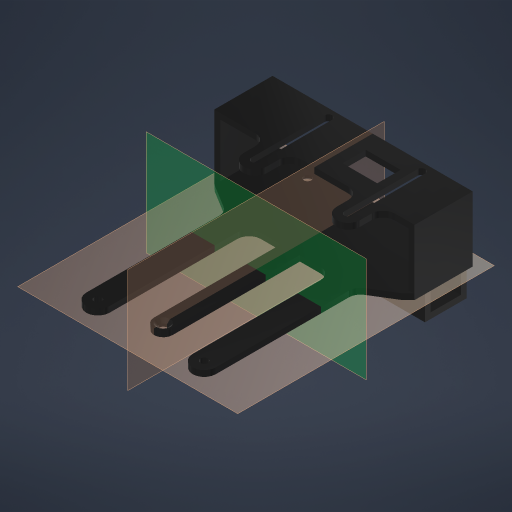
# Autodesk Inventor part: PD_Main
Saved by Autodesk Inventor 2024 (Build 280153000, 153)
## iProperties
Manager: Louis Van Roosmaelen
Company: DCS - DIGITAL COMBAT SIMULATOR
Created: 2023-12-17
Part Number: PD_Main
Material: S235
Catalog Web Link: http://emmausbovenbouw.op-weg.be/
Vendor: Emmaüsinstituut Bovenbouw Aalter
Document SubType Name: Modeling
Designer: Louis
Engineer: Declercq St.
Manufacturer: Standard
Standards Organization: Custom
Density: 7.86 g/cm^3
Appearance: Smooth - Black
Mass: 188.232 g
Surface Area: 215.295 cm^2
Volume: 23.9481 cm^3
IDENT.NR.: AJ2022
TEAM: 30
Title: F18C Home Cockpit
Author: Louis
Keywords: Ø
Autodesk Inventor part; units mm, degrees
sketch "Sketch1" plane through (0, 0, 0) normal (0, 0, 1) x (1, 0, 0)
  line L0 (0, 2.8582) -> (0, -2.8582) construction
  line L1 (-5.7775, 0) -> (5.7775, 0) construction
  line L2 (-40.5, -50) -> (40.5, -50)
  line L3 (40.5, -50) -> (40.5, 50)
  line L4 (40.5, 50) -> (-40.5, 50)
  line L5 (-40.5, 50) -> (-40.5, -50)
  line L6 (-40.5, -50) -> (40.5, 50) construction
  line L7 (40.5, -50) -> (-40.5, 50) construction
  line L8 (-43, 52.5) -> (43, 52.5)
  line L9 (43, 52.5) -> (43, -52.5)
  line L10 (43, -52.5) -> (-43, -52.5)
  line L11 (-43, -52.5) -> (-43, 52.5)
  line L12 (-43, 52.5) -> (43, -52.5) construction
  line L13 (43, 52.5) -> (-43, -52.5) construction
  point P0 (0, 0)
  point P1 (0, 0)
  dimension "d0" = 81
  dimension "d1" = 100
  dimension "d2" = 2.5
  dimension "d3" = 2.5
  constraints: 28 end point, 6 midpoint, 4 parallel, 3 horizontal, 2 perpendicular, 1 coincident, 1 vertical
  measures "d0" distance of L4.end L3.end
  measures "d1" distance of L3.end L2.end
  measures "d2" distance between parallel lines of L3 L9
  measures "d3" distance between parallel lines of L10 L2
extrude "Extrusion1" add sketch "Sketch1" along normal blind 2.5 contours L5 L4 L3 L2
sketch "Sketch2" plane through (0, 0, 0) normal (0, 0, -1) x (-1, 0, 0)
  line L0 (40.5, -50) -> (-40.5, -50) projected
  line L1 (-40.5, -50) -> (-40.5, 50) projected
  line L2 (-40.5, 50) -> (40.5, 50) projected
  line L3 (40.5, 50) -> (40.5, -50) projected
  line L4 (-40.5, 50) -> (-13, 50)
  line L5 (-13, 50) -> (-13, 32)
  line L6 (-13, 32) -> (-40.5, 32)
  line L7 (-40.5, 32) -> (-40.5, 50)
  line L8 (-40.5, 34.5) -> (-15.5, 34.5)
  line L9 (-15.5, 34.5) -> (-15.5, 47.5)
  line L10 (-15.5, 47.5) -> (-40.5, 47.5)
  point P0 (0, 0)
  dimension "d6" = 27.5
  dimension "d7" = 18
  dimension "d8" = 2.5
  dimension "d9" = 2.5
  dimension "d10" = 2.5
  constraints: 14 end point, 3 perpendicular, 2 parallel, 2 point on line, 1 horizontal, 1 vertical
  measures "d6" distance of L5.end L6.end
  measures "d7" distance of L4.end L5.end
  measures "d8" distance between parallel lines of L2 L10
  measures "d9" distance between parallel lines of L6 L8
  measures "d10" distance between parallel lines of L5 L9
extrude "Extrusion2" add sketch "Sketch2" along normal blind 13 contours L1 L8 L9 L10 L2 L5 L6
sketch "Sketch3" plane through (0, 0, -13) normal (0, 0, -1) x (-1, 0, 0)
  line L0 (-13, 50) -> (-13, 32) projected
  line L1 (-13, 32) -> (-40.5, 32) projected
  line L2 (-40.5, 32) -> (-40.5, 34.5) projected
  line L3 (-40.5, 34.5) -> (-15.5, 34.5) projected
  line L4 (-15.5, 34.5) -> (-15.5, 47.5) projected
  line L5 (-15.5, 47.5) -> (-40.5, 47.5) projected
  line L6 (-40.5, 47.5) -> (-40.5, 50) projected
  line L7 (-40.5, 50) -> (-13, 50) projected
  line L8 (-40.5, 34.5) -> (-40.5, 47.5) projected
  line L9 (-40.5, 34.5) -> (-40.5, 47.5)
  point P0 (0, 0)
  constraints: 2 end point, 1 vertical
extrude "Extrusion3" add sketch "Sketch3" against normal blind 2.5 contours L5 L4 L3 L8
sketch "Sketch4" plane through (13, 32, 0) normal (-1, 0, 0) x (0, 0, 1)
  line L0 (0, 18) -> (0, 0) projected
  line L1 (0, 0) -> (-13, 0) projected
  line L2 (-13, 0) -> (-13, 18) projected
  line L3 (-13, 18) -> (0, 18) projected
  line L4 (0, 18) -> (2.5, 18) projected
  line L5 (2.5, 18) -> (2.5, -82) projected
  line L6 (2.5, -82) -> (0, -82) projected
  line L7 (0, -82) -> (0, 0) projected
  point P0 (0, -32)
  point P1 (-5.25, 11)
  point P2 (-5.25, 7)
  dimension "d15" = 7
  dimension "d16" = 4
  dimension "d19" = 5.25
  dimension "d20" = 5.25
  measures "d15" distance from line of point (-5.25, 7) L1
  measures "d16" distance of point (-5.25, 7) point (-5.25, 11)
  measures "d19" distance from line of L0 point (-5.25, 7)
  measures "d20" distance from line of L0 point (-5.25, 11)
hole "Hole1" at (13, 43, -5.25) at (13, 39, -5.25) direction (1, 0, 0) diameter 4 end through all counterbore diameter 8 counterbore depth 4
sketch "Sketch6" plane through (40.5, -50, 2.5) normal (1, 0, 0) x (0, 0, -1)
  line L0 (13, 84.5) -> (13, 97.5) projected
  line L1 (13, 97.5) -> (2.5, 97.5) projected
  line L2 (2.5, 97.5) -> (2.5, 84.5) projected
  line L3 (2.5, 84.5) -> (13, 84.5) projected
  line L4 (15.5, 82) -> (2.5, 82) projected
  line L5 (2.5, 82) -> (2.5, 0) projected
  line L6 (2.5, 0) -> (0, 0) projected
  line L7 (0, 0) -> (0, 100) projected
  line L8 (0, 100) -> (15.5, 100) projected
  line L9 (15.5, 100) -> (15.5, 82) projected
  line L10 (2.5, 100) -> (2.5, 82) projected
  line L11 (2.5, 100) -> (-25.5, 100)
  line L12 (-25.5, 100) -> (-25.5, 75)
  line L13 (-25.5, 75) -> (2.5, 75)
  line L14 (2.5, 75) -> (2.5, 100)
  point P0 (2.5, 50)
  dimension "d32" = 28
  dimension "d33" = 25
  constraints: 8 end point, 2 parallel, 1 horizontal, 1 perpendicular
  measures "d32" distance of L13.end L12.end
  measures "d33" distance of L12.end L11.end
extrude "Extrusion5" add sketch "Sketch6" along normal blind 2.5 contours L10 L5 L13 L7 L8 L2 | L7 L13 L12 L11
mirror "Mirror2" about plane through (0, 0, 0) normal (1, 0, 0) of "Extrusion5", "Hole1", "Extrusion3", "Extrusion2"
sketch "Sketch7" plane through (40.5, 25, 28) normal (0, 0, 1) x (1, 0, 0)
  line L0 (-81, 25) -> (-81, 0) projected
  line L1 (-81, 0) -> (-83.5, 0) projected
  line L2 (-83.5, 0) -> (-83.5, 25) projected
  line L3 (-83.5, 25) -> (-81, 25) projected
  line L4 (0, 0) -> (0, 25) projected
  line L5 (0, 25) -> (2.5, 25) projected
  line L6 (2.5, 25) -> (2.5, 0) projected
  line L7 (2.5, 0) -> (0, 0) projected
  line L8 (0, 0) -> (-81, 0)
  line L9 (-81, 25) -> (0, 25)
  point P0 (-40.5, -25)
  constraints: 4 end point, 1 horizontal, 1 parallel
extrude "Extrusion6" add sketch "Sketch7" against normal blind 2.5 contours L9 L4 L8 L0
chamfer "Chamfer1" distance 2.5 angle 45 2 edges at (-40.5, 25, 1.25) (40.5, 25, 1.25)
sketch "Sketch9" plane through (0, 0, 2.5) normal (0, 0, 1) x (1, 0, 0)
  line L0 (-40.5, 22.5) -> (-43, 25) projected
  line L1 (-40.5, 25) -> (-43, 25) projected
  line L2 (-40.5, 50) -> (-40.5, 25) projected
  line L3 (-43, 50) -> (-40.5, 50) projected
  line L4 (-43, 25) -> (-43, 50) projected
  line L5 (-40.5, -50) -> (-40.5, 22.5) projected
  line L6 (40.5, -50) -> (-40.5, -50) projected
  line L7 (40.5, 22.5) -> (40.5, -50) projected
  line L8 (43, 25) -> (40.5, 22.5) projected
  line L9 (43, 50) -> (43, 25) projected
  line L10 (40.5, 50) -> (43, 50) projected
  line L11 (-40.5, 50) -> (40.5, 50) projected
  line L12 (43, 25) -> (40.5, 25) projected
  line L13 (40.5, 25) -> (40.5, 50) projected
  circle A0 centre (-22.86, -45.25) radius 5
  circle A1 centre (22.86, -45.25) radius 5
  line L14 (-27.86, -45.25) -> (-27.86, 14.75)
  line L15 (-27.86, 14.75) -> (-40.5, 22.5)
  line L16 (-17.86, -45.25) -> (-17.86, 14.75)
  line L17 (-17.86, -45.25) -> (42.14, -45.25) construction
  line L18 (17.86, -45.25) -> (17.86, 14.75)
  line L19 (17.86, 14.75) -> (-17.86, 14.75)
  line L20 (27.86, -45.25) -> (27.86, 14.75)
  line L21 (27.86, 14.75) -> (40.5, 22.5)
  point P0 (0, 0)
  point P1 (24.4212, -50)
  point P2 (-21.2988, -50)
  point P3 (21.2988, -50)
  point P4 (-24.4212, -50)
  dimension "d58" = 10
  dimension "d59" = 10
  dimension "d60" = 60
  dimension "d61" = 60
  dimension "d62" = 90
  dimension "d63" = 60
  dimension "d64" = 60
  dimension "d65" = 90
  constraints: 16 end point, 4 point on circle, 3 point on line, 2 centre point, 2 coincident, 2 perpendicular, 2 tangent, 1 horizontal, 1 parallel, 1 vertical
  measures "d58" diameter of A0
  measures "d59" diameter of A1
  measures "d60" distance of L14.start L14.end
  measures "d61" distance of L16.start L16.end
  measures "d62" angle of L17 L16
  measures "d63" distance of L18.start L18.end
  measures "d64" distance of L20.start L20.end
  measures "d65" angle of L17 L20
extrude "Extrusion7" cut sketch "Sketch9" against normal up to surface (2.5 mm away) contours L15 L14 A0 L6 L5 | A0 L16 L19 L18 A1 L6 | A1 L20 L21 L7 L6
sketch "Sketch10" plane through (43, 25, 28) normal (0, 0, 1) x (1, 0, 0)
  line L0 (0, 0) -> (-86, 0) projected
  line L1 (-86, 0) -> (-86, 25) projected
  line L2 (-86, 25) -> (0, 25) projected
  line L3 (0, 25) -> (0, 0) projected
  circle A0 centre (-58.5, -10) radius 1.65
  circle A1 centre (-58.5, 21.5) radius 1.65
  circle A2 centre (-18.5, -10) radius 1.65
  circle A3 centre (-18.5, 21.5) radius 1.65
  line L4 (-60.15, -10) -> (-60.15, 21.5)
  line L5 (-56.85, -10) -> (-56.85, 21.5)
  line L6 (-20.15, -10) -> (-20.15, 21.5)
  line L7 (-16.85, -10) -> (-16.85, 21.5)
  circle A4 centre (-58.5, -10) radius 5
  circle A5 centre (-58.5, 21.5) radius 5
  circle A6 centre (-18.5, 21.5) radius 5
  circle A7 centre (-18.5, -10) radius 5
  line L8 (-63.5, -10) -> (-63.5, 21.5)
  line L9 (-53.5, -10) -> (-53.5, 21.5)
  line L10 (-13.5, 21.5) -> (-13.5, -10)
  line L11 (-23.5, -10) -> (-23.5, 21.5)
  point P0 (-43, -25)
  point P1 (-23.5, 0)
  point P2 (-13.5, 0)
  point P3 (-63.5, 0)
  point P4 (-53.5, 0)
  dimension "d68" = 3.3
  dimension "d69" = 3.3
  dimension "d70" = 3.3
  dimension "d71" = 3.3
  dimension "d74" = 40
  dimension "d75" = 40
  dimension "d76" = 15.5
  dimension "d77" = 24.5
  dimension "d78" = 10
  dimension "d79" = 10
  dimension "d80" = 10
  dimension "d81" = 10
  dimension "d82" = 35
  dimension "d83" = 35
  dimension "d88" = 3.5
  dimension "d89" = 3.5
  constraints: 16 end point, 16 point on circle, 8 centre point, 7 tangent, 4 coincident, 2 vertical, 1 parallel
  measures "d68" diameter of A0
  measures "d69" diameter of A1
  measures "d70" diameter of A2
  measures "d71" diameter of A3
  measures "d74" distance of A1.centre A3.centre
  measures "d75" distance of A2.centre A0.centre
  measures "d76" horizontal distance of point (-43, -25) A1.centre
  measures "d77" horizontal distance of point (-43, -25) A2.centre
  measures "d78" diameter of A4
  measures "d79" diameter of A5
  measures "d80" diameter of A6
  measures "d81" diameter of A7
  measures "d82" distance from line of L2 A0.centre
  measures "d83" distance from line of L2 A2.centre
  measures "d88" distance from line of L2 A1.centre
  measures "d89" distance from line of L2 A3.centre
extrude "Extrusion8" add sketch "Sketch10" against normal up to surface (2.5 mm away) contours L10 A7 L7 L0 | L7 A7 L6 L0 | A7 L6 A2 L7 | L6 A7 L11 L0 | L7 A2 L6 A7 | L9 A4 L5 L0 | L5 A4 L4 L0 | A4 L4 A0 L5 | L4 A4 L8 L0 | L5 A0 L4 A4
extrude "Extrusion9" cut sketch "Sketch10" against normal up to surface (2.5 mm away) contours L7 A7 L6 L0 | L0 L6 A6 L7 | L7 A2 L6 A7 | A6 L6 A3 L7 | A3 | L5 A4 L4 L0 | L0 L4 A5 L5 | A5 L4 A1 L5 | L5 A0 L4 A4 | A1 picked at (-18.4337, -6.1416) picked at (-58.5663, -6.1416)
fillet "Fillet1" radius 5 9 edges at (-17.86, 14.75, 1.25) (17.86, 14.75, 1.25) (27.86, 14.75, 1.25) (-27.86, 14.75, 1.25) (-40.5, 22.5001, 1.25) (29.5, 25, 26.75) (19.5, 25, 26.75) (-10.5, 25, 26.75) (-20.5, 25, 26.75)
sketch "Sketch11" plane through (0, 0, 0) normal (0, 0, -1) x (-1, 0, 0)
  arc A0 (24.4212, -50) -> (27.86, -45.25) centre (22.86, -45.25) ccw projected
  line L0 (24.4212, -50) -> (21.2988, -50) projected
  arc A1 (17.86, -45.25) -> (21.2988, -50) centre (22.86, -45.25) ccw projected
  line L1 (17.86, -45.25) -> (17.86, 9.75) projected
  arc A2 (17.86, 9.75) -> (12.86, 14.75) centre (12.86, 9.75) ccw projected
  line L2 (12.86, 14.75) -> (-12.86, 14.75) projected
  arc A3 (-12.86, 14.75) -> (-17.86, 9.75) centre (-12.86, 9.75) ccw projected
  line L3 (-17.86, 9.75) -> (-17.86, -45.25) projected
  arc A4 (-21.2988, -50) -> (-17.86, -45.25) centre (-22.86, -45.25) ccw projected
  line L4 (-21.2988, -50) -> (-24.4212, -50) projected
  arc A5 (-27.86, -45.25) -> (-24.4212, -50) centre (-22.86, -45.25) ccw projected
  line L5 (-27.86, -45.25) -> (-27.86, 11.9507) projected
  arc A6 (-27.86, 11.9507) -> (-30.2465, 16.2132) centre (-32.86, 11.9507) ccw projected
  line L6 (-30.2465, 16.2132) -> (-40.5, 22.5) projected
  line L7 (-40.5, 22.5) -> (-43, 25) projected
  line L8 (-43, 25) -> (-43, 50) projected
  line L9 (-43, 50) -> (-40.5, 50) projected
  line L10 (-40.5, 50) -> (-13, 50) projected
  line L11 (-13, 32) -> (-13, 50) projected
  line L12 (-40.5, 32) -> (-13, 32) projected
  line L13 (-40.5, 34.5) -> (-40.5, 32) projected
  line L14 (-15.5, 34.5) -> (-40.5, 34.5) projected
  line L15 (-15.5, 47.5) -> (-15.5, 34.5) projected
  line L16 (-40.5, 47.5) -> (-15.5, 47.5) projected
  line L17 (-40.5, 50) -> (-40.5, 47.5) projected
  line L18 (27.86, 11.9507) -> (27.86, -45.25) projected
  arc A7 (30.2465, 16.2132) -> (27.86, 11.9507) centre (32.86, 11.9507) ccw projected
  line L19 (39.996, 22.191) -> (30.2465, 16.2132) projected
  arc A8 (39.996, 22.191) -> (40.918, 22.918) centre (37.3825, 26.4536) ccw projected
  line L20 (43, 25) -> (40.918, 22.918) projected
  line L21 (43, 50) -> (43, 25) projected
  line L22 (40.5, 50) -> (43, 50) projected
  line L23 (13, 50) -> (40.5, 50) projected
  line L24 (13, 50) -> (13, 32) projected
  line L25 (13, 32) -> (40.5, 32) projected
  line L26 (40.5, 32) -> (40.5, 34.5) projected
  line L27 (40.5, 34.5) -> (15.5, 34.5) projected
  line L28 (15.5, 34.5) -> (15.5, 47.5) projected
  line L29 (15.5, 47.5) -> (40.5, 47.5) projected
  line L30 (40.5, 47.5) -> (40.5, 50) projected
  line L31 (-13, 50) -> (13, 50) projected
  point P0 (0, 0)
  point P1 (-22.86, 44.92)
  point P2 (22.86, 44.92)
  dimension "d106" = 90.17
  dimension "d107" = 90.17
  dimension "d108" = 45.72
  dimension "d109" = 45.72
  dimension "d110" = 45.72
  constraints: 2 coincident
  measures "d106" distance of point (-22.86, -45.25) point (-22.86, 44.92)
  measures "d107" distance of point (22.86, -45.25) point (22.86, 44.92)
  measures "d108" distance of point (22.86, 44.92) point (-22.86, 44.92)
  measures "d109" distance of point (22.86, -45.25) point (-22.86, -45.25)
  measures "d110" horizontal distance of A0.centre point (-22.86, 44.92)
hole "Hole3" at (22.86, 44.92, 0) at (-22.86, 44.92, 0) direction (0, 0, 1) diameter 3.3 depth 2.5 countersink diameter 6 countersink angle 90
sketch "Sketch12" plane through (0, 0, 0) normal (0, 0, -1) x (-1, 0, 0)
  arc A0 (-24.3909, 47.5) -> (-21.3291, 47.5) centre (-22.86, 44.92) ccw projected
  arc A1 (-24.3909, 47.5) -> (-21.3291, 47.5) centre (-22.86, 44.92) ccw projected
  arc A2 (-21.3291, 47.5) -> (-24.3909, 47.5) centre (-22.86, 44.92) ccw projected
  circle A3 centre (-22.86, 44.92) radius 1.65 projected
  arc A4 (21.3291, 47.5) -> (24.3909, 47.5) centre (22.86, 44.92) ccw projected
  arc A5 (24.3909, 47.5) -> (21.3291, 47.5) centre (22.86, 44.92) ccw projected
  circle A6 centre (22.86, 44.92) radius 1.65 projected
  arc A7 (24.4212, -50) -> (27.86, -45.25) centre (22.86, -45.25) ccw projected
  line L0 (24.4212, -50) -> (21.2988, -50) projected
  arc A8 (17.86, -45.25) -> (21.2988, -50) centre (22.86, -45.25) ccw projected
  line L1 (17.86, -45.25) -> (17.86, 9.75) projected
  arc A9 (17.86, 9.75) -> (12.86, 14.75) centre (12.86, 9.75) ccw projected
  line L2 (12.86, 14.75) -> (-12.86, 14.75) projected
  arc A10 (-12.86, 14.75) -> (-17.86, 9.75) centre (-12.86, 9.75) ccw projected
  line L3 (-17.86, 9.75) -> (-17.86, -45.25) projected
  arc A11 (-21.2988, -50) -> (-17.86, -45.25) centre (-22.86, -45.25) ccw projected
  line L4 (-21.2988, -50) -> (-24.4212, -50) projected
  arc A12 (-27.86, -45.25) -> (-24.4212, -50) centre (-22.86, -45.25) ccw projected
  line L5 (-27.86, -45.25) -> (-27.86, 11.9507) projected
  arc A13 (-27.86, 11.9507) -> (-30.2465, 16.2132) centre (-32.86, 11.9507) ccw projected
  line L6 (-30.2465, 16.2132) -> (-40.5, 22.5) projected
  line L7 (-40.5, 22.5) -> (-43, 25) projected
  line L8 (-43, 25) -> (-43, 50) projected
  line L9 (-43, 50) -> (-40.5, 50) projected
  line L10 (-40.5, 50) -> (-13, 50) projected
  line L11 (-13, 32) -> (-13, 50) projected
  line L12 (-40.5, 32) -> (-13, 32) projected
  line L13 (-40.5, 34.5) -> (-40.5, 32) projected
  line L14 (-15.5, 34.5) -> (-40.5, 34.5) projected
  line L15 (-15.5, 47.5) -> (-15.5, 34.5) projected
  line L16 (-21.3291, 47.5) -> (-15.5, 47.5) projected
  arc A14 (-21.3291, 47.5) -> (-24.3909, 47.5) centre (-22.86, 44.92) ccw projected
  line L17 (-40.5, 47.5) -> (-24.3909, 47.5) projected
  line L18 (-40.5, 50) -> (-40.5, 47.5) projected
  line L19 (27.86, 11.9507) -> (27.86, -45.25) projected
  arc A15 (30.2465, 16.2132) -> (27.86, 11.9507) centre (32.86, 11.9507) ccw projected
  line L20 (39.996, 22.191) -> (30.2465, 16.2132) projected
  arc A16 (39.996, 22.191) -> (40.918, 22.918) centre (37.3825, 26.4536) ccw projected
  line L21 (43, 25) -> (40.918, 22.918) projected
  line L22 (43, 50) -> (43, 25) projected
  line L23 (40.5, 50) -> (43, 50) projected
  line L24 (13, 50) -> (40.5, 50) projected
  line L25 (13, 50) -> (13, 32) projected
  line L26 (13, 32) -> (40.5, 32) projected
  line L27 (40.5, 32) -> (40.5, 34.5) projected
  line L28 (40.5, 34.5) -> (15.5, 34.5) projected
  line L29 (15.5, 34.5) -> (15.5, 47.5) projected
  line L30 (15.5, 47.5) -> (21.3291, 47.5) projected
  arc A17 (24.3909, 47.5) -> (21.3291, 47.5) centre (22.86, 44.92) ccw projected
  line L31 (24.3909, 47.5) -> (40.5, 47.5) projected
  line L32 (40.5, 47.5) -> (40.5, 50) projected
  line L33 (-13, 50) -> (13, 50) projected
  arc A18 (-24.3909, 47.5) -> (-21.3291, 47.5) centre (-22.86, 44.92) ccw projected
  line L34 (-21.3291, 47.5) -> (-24.3909, 47.5) projected
  arc A19 (21.3291, 47.5) -> (24.3909, 47.5) centre (22.86, 44.92) ccw projected
  line L35 (24.3909, 47.5) -> (21.3291, 47.5) projected
  arc A20 (24.4212, -50) -> (27.86, -45.25) centre (22.86, -45.25) ccw projected
  line L36 (24.4212, -50) -> (21.2988, -50) projected
  arc A21 (17.86, -45.25) -> (21.2988, -50) centre (22.86, -45.25) ccw projected
  line L37 (17.86, -45.25) -> (17.86, 9.75) projected
  arc A22 (17.86, 9.75) -> (12.86, 14.75) centre (12.86, 9.75) ccw projected
  line L38 (12.86, 14.75) -> (-12.86, 14.75) projected
  arc A23 (-12.86, 14.75) -> (-17.86, 9.75) centre (-12.86, 9.75) ccw projected
  line L39 (-17.86, 9.75) -> (-17.86, -45.25) projected
  arc A24 (-21.2988, -50) -> (-17.86, -45.25) centre (-22.86, -45.25) ccw projected
  line L40 (-21.2988, -50) -> (-24.4212, -50) projected
  arc A25 (-27.86, -45.25) -> (-24.4212, -50) centre (-22.86, -45.25) ccw projected
  line L41 (-27.86, -45.25) -> (-27.86, 11.9507) projected
  arc A26 (-27.86, 11.9507) -> (-30.2465, 16.2132) centre (-32.86, 11.9507) ccw projected
  line L42 (-30.2465, 16.2132) -> (-40.5, 22.5) projected
  line L43 (-40.5, 22.5) -> (-43, 25) projected
  line L44 (-43, 25) -> (-43, 50) projected
  line L45 (-43, 50) -> (-40.5, 50) projected
  line L46 (-40.5, 50) -> (-13, 50) projected
  line L47 (-13, 32) -> (-13, 50) projected
  line L48 (-40.5, 32) -> (-13, 32) projected
  line L49 (-40.5, 34.5) -> (-40.5, 32) projected
  line L50 (-15.5, 34.5) -> (-40.5, 34.5) projected
  line L51 (-15.5, 47.5) -> (-15.5, 34.5) projected
  line L52 (-21.3291, 47.5) -> (-15.5, 47.5) projected
  arc A27 (-21.3291, 47.5) -> (-24.3909, 47.5) centre (-22.86, 44.92) ccw projected
  line L53 (-40.5, 47.5) -> (-24.3909, 47.5) projected
  line L54 (-40.5, 50) -> (-40.5, 47.5) projected
  line L55 (27.86, 11.9507) -> (27.86, -45.25) projected
  arc A28 (30.2465, 16.2132) -> (27.86, 11.9507) centre (32.86, 11.9507) ccw projected
  line L56 (39.996, 22.191) -> (30.2465, 16.2132) projected
  arc A29 (39.996, 22.191) -> (40.918, 22.918) centre (37.3825, 26.4536) ccw projected
  line L57 (43, 25) -> (40.918, 22.918) projected
  line L58 (43, 50) -> (43, 25) projected
  line L59 (40.5, 50) -> (43, 50) projected
  line L60 (13, 50) -> (40.5, 50) projected
  line L61 (13, 50) -> (13, 32) projected
  line L62 (13, 32) -> (40.5, 32) projected
  line L63 (40.5, 32) -> (40.5, 34.5) projected
  line L64 (40.5, 34.5) -> (15.5, 34.5) projected
  line L65 (15.5, 34.5) -> (15.5, 47.5) projected
  line L66 (15.5, 47.5) -> (21.3291, 47.5) projected
  arc A30 (24.3909, 47.5) -> (21.3291, 47.5) centre (22.86, 44.92) ccw projected
  line L67 (24.3909, 47.5) -> (40.5, 47.5) projected
  line L68 (40.5, 47.5) -> (40.5, 50) projected
  line L69 (-13, 50) -> (13, 50) projected
  arc A31 (-24.3909, 47.5) -> (-21.3291, 47.5) centre (-22.86, 44.92) ccw projected
  line L70 (-21.3291, 47.5) -> (-24.3909, 47.5) projected
  arc A32 (21.3291, 47.5) -> (24.3909, 47.5) centre (22.86, 44.92) ccw projected
  line L71 (24.3909, 47.5) -> (21.3291, 47.5) projected
  point P0 (0, 0)
  point P1 (-21.3291, 47.5)
extrude "Extrusion10" cut sketch "Sketch12" along normal up to surface (13 mm away) contours L34 A0 | A2 L34 | L35 A5 | A4 L35 | A3 | A6
sketch "Sketch13" plane through (0, 0, 0) normal (0, 0, -1) x (-1, 0, 0)
  arc A0 (24.4212, -50) -> (27.86, -45.25) centre (22.86, -45.25) ccw projected
  line L0 (24.4212, -50) -> (21.2988, -50) projected
  arc A1 (17.86, -45.25) -> (21.2988, -50) centre (22.86, -45.25) ccw projected
  line L1 (17.86, -45.25) -> (17.86, 9.75) projected
  arc A2 (17.86, 9.75) -> (12.86, 14.75) centre (12.86, 9.75) ccw projected
  line L2 (12.86, 14.75) -> (-12.86, 14.75) projected
  arc A3 (-12.86, 14.75) -> (-17.86, 9.75) centre (-12.86, 9.75) ccw projected
  line L3 (-17.86, 9.75) -> (-17.86, -45.25) projected
  arc A4 (-21.2988, -50) -> (-17.86, -45.25) centre (-22.86, -45.25) ccw projected
  line L4 (-21.2988, -50) -> (-24.4212, -50) projected
  arc A5 (-27.86, -45.25) -> (-24.4212, -50) centre (-22.86, -45.25) ccw projected
  line L5 (-27.86, -45.25) -> (-27.86, 11.9507) projected
  arc A6 (-27.86, 11.9507) -> (-30.2465, 16.2132) centre (-32.86, 11.9507) ccw projected
  line L6 (-30.2465, 16.2132) -> (-40.5, 22.5) projected
  line L7 (-40.5, 22.5) -> (-43, 25) projected
  line L8 (-43, 25) -> (-43, 50) projected
  line L9 (-43, 50) -> (-40.5, 50) projected
  line L10 (-40.5, 50) -> (-13, 50) projected
  line L11 (-13, 32) -> (-13, 50) projected
  line L12 (-40.5, 32) -> (-13, 32) projected
  line L13 (-40.5, 34.5) -> (-40.5, 32) projected
  line L14 (-15.5, 34.5) -> (-40.5, 34.5) projected
  line L15 (-15.5, 47.5) -> (-15.5, 34.5) projected
  line L16 (-21.3291, 47.5) -> (-15.5, 47.5) projected
  arc A7 (-24.3909, 47.5) -> (-21.3291, 47.5) centre (-22.86, 44.92) ccw projected
  arc A8 (-21.3291, 47.5) -> (-24.3909, 47.5) centre (-22.86, 44.92) ccw projected
  line L17 (27.86, 11.9507) -> (27.86, -45.25) projected
  arc A9 (30.2465, 16.2132) -> (27.86, 11.9507) centre (32.86, 11.9507) ccw projected
  line L18 (39.996, 22.191) -> (30.2465, 16.2132) projected
  arc A10 (39.996, 22.191) -> (40.918, 22.918) centre (37.3825, 26.4536) ccw projected
  line L19 (43, 25) -> (40.918, 22.918) projected
  line L20 (43, 50) -> (43, 25) projected
  line L21 (40.5, 50) -> (43, 50) projected
  line L22 (13, 50) -> (40.5, 50) projected
  line L23 (13, 50) -> (13, 32) projected
  line L24 (13, 32) -> (40.5, 32) projected
  line L25 (40.5, 32) -> (40.5, 34.5) projected
  line L26 (40.5, 34.5) -> (15.5, 34.5) projected
  line L27 (15.5, 34.5) -> (15.5, 47.5) projected
  line L28 (21.3291, 47.5) -> (15.5, 47.5) projected
  arc A11 (21.3291, 47.5) -> (24.3909, 47.5) centre (22.86, 44.92) ccw projected
  line L29 (24.3909, 47.5) -> (40.5, 47.5) projected
  line L30 (40.5, 47.5) -> (40.5, 50) projected
  line L31 (-40.5, 50) -> (-40.5, 47.5) projected
  line L32 (-24.3909, 47.5) -> (-40.5, 47.5) projected
  line L33 (-13, 50) -> (13, 50) projected
  arc A12 (24.3909, 47.5) -> (21.3291, 47.5) centre (22.86, 44.92) ccw projected
  circle A13 centre (0, -40) radius 4
  line L34 (4, -40) -> (4, 14.75)
  line L35 (-4, -40) -> (-4, 14.75)
  point P0 (0, 0)
  dimension "d120" = 90
  dimension "d121" = 8
  dimension "d122" = 0
  constraints: 4 end point, 2 point on circle, 2 point on line, 2 tangent, 1 centre point, 1 coincident, 1 perpendicular, 1 vertical
  measures "d120" distance from line of L33 point (0, -40)
  measures "d121" diameter of A13
  measures "d122" horizontal distance of point (0, 0) point (0, -40)
extrude "Extrusion11" add sketch "Sketch13" against normal up to surface (2.5 mm away) contours L34 A13 L35 L2 | A13
sketch "Sketch14" plane through (0, 0, 2.5) normal (0, 0, 1) x (1, 0, 0)
  circle A0 centre (-22.86, 44.92) radius 1.65 projected
  circle A1 centre (22.86, 44.92) radius 1.65 projected
  arc A2 (-40.918, 22.918) -> (-39.996, 22.191) centre (-37.3825, 26.4536) ccw projected
  line L0 (-40.918, 22.918) -> (-43, 25) projected
  line L1 (-43, 25) -> (-40.5, 25) projected
  line L2 (-40.5, 25) -> (-40.5, 50) projected
  line L3 (-40.5, 50) -> (40.5, 50) projected
  line L4 (40.5, 50) -> (40.5, 25) projected
  line L5 (40.5, 25) -> (43, 25) projected
  line L6 (43, 25) -> (40.5, 22.5) projected
  line L7 (40.5, 22.5) -> (30.2465, 16.2132) projected
  arc A3 (30.2465, 16.2132) -> (27.86, 11.9507) centre (32.86, 11.9507) ccw projected
  line L8 (27.86, 11.9507) -> (27.86, -45.25) projected
  arc A4 (24.4212, -50) -> (27.86, -45.25) centre (22.86, -45.25) ccw projected
  line L9 (24.4212, -50) -> (21.2988, -50) projected
  arc A5 (17.86, -45.25) -> (21.2988, -50) centre (22.86, -45.25) ccw projected
  line L10 (17.86, -45.25) -> (17.86, 9.75) projected
  arc A6 (17.86, 9.75) -> (12.86, 14.75) centre (12.86, 9.75) ccw projected
  line L11 (12.86, 14.75) -> (4, 14.75) projected
  line L12 (4, 14.75) -> (4, -40) projected
  arc A7 (-4, -40) -> (4, -40) centre (0, -40) ccw projected
  line L13 (-4, -40) -> (-4, 14.75) projected
  line L14 (-4, 14.75) -> (-12.86, 14.75) projected
  arc A8 (-12.86, 14.75) -> (-17.86, 9.75) centre (-12.86, 9.75) ccw projected
  line L15 (-17.86, 9.75) -> (-17.86, -45.25) projected
  arc A9 (-21.2988, -50) -> (-17.86, -45.25) centre (-22.86, -45.25) ccw projected
  line L16 (-21.2988, -50) -> (-24.4212, -50) projected
  arc A10 (-27.86, -45.25) -> (-24.4212, -50) centre (-22.86, -45.25) ccw projected
  line L17 (-27.86, -45.25) -> (-27.86, 11.9507) projected
  arc A11 (-27.86, 11.9507) -> (-30.2465, 16.2132) centre (-32.86, 11.9507) ccw projected
  line L18 (-30.2465, 16.2132) -> (-39.996, 22.191) projected
  line L19 (-43, 25) -> (-43, 50) projected
  line L20 (-43, 50) -> (-40.5, 50) projected
  line L21 (40.5, 50) -> (43, 50) projected
  line L22 (43, 50) -> (43, 25) projected
  point P0 (0, 0)
  constraints: 1 coincident
hole "Hole4" at (0, -40, 2.5) direction (0, 0, -1) diameter 3.3 depth 2.5 countersink diameter 6 countersink angle 90
sketch "Sketch15" plane through (43, 25, 28) normal (0, 0, 1) x (1, 0, 0)
  arc A0 (-8.5, 0) -> (-13.5, -5) centre (-8.5, -5) ccw projected
  line L0 (-13.5, -5) -> (-13.5, -10) projected
  arc A1 (-23.5, -10) -> (-13.5, -10) centre (-18.5, -10) ccw projected
  line L1 (-23.5, -10) -> (-23.5, -5) projected
  arc A2 (-23.5, -5) -> (-28.5, 0) centre (-28.5, -5) ccw projected
  line L2 (-28.5, 0) -> (-48.5, 0) projected
  arc A3 (-48.5, 0) -> (-53.5, -5) centre (-48.5, -5) ccw projected
  line L3 (-53.5, -5) -> (-53.5, -10) projected
  arc A4 (-63.5, -10) -> (-53.5, -10) centre (-58.5, -10) ccw projected
  line L4 (-63.5, -10) -> (-63.5, -5) projected
  arc A5 (-63.5, -5) -> (-68.5, 0) centre (-68.5, -5) ccw projected
  line L5 (-68.5, 0) -> (-86, 0) projected
  line L6 (-86, 0) -> (-86, 25) projected
  line L7 (-86, 25) -> (0, 25) projected
  line L8 (0, 25) -> (0, 0) projected
  line L9 (0, 0) -> (-8.5, 0) projected
  line L10 (-56.85, -10) -> (-56.85, 21.5) projected
  arc A6 (-56.85, 21.5) -> (-60.15, 21.5) centre (-58.5, 21.5) ccw projected
  line L11 (-60.15, 21.5) -> (-60.15, -10) projected
  arc A7 (-60.15, -10) -> (-56.85, -10) centre (-58.5, -10) ccw projected
  line L12 (-20.15, 21.5) -> (-20.15, -10) projected
  arc A8 (-20.15, -10) -> (-16.85, -10) centre (-18.5, -10) ccw projected
  line L13 (-16.85, -10) -> (-16.85, 21.5) projected
  arc A9 (-16.85, 21.5) -> (-20.15, 21.5) centre (-18.5, 21.5) ccw projected
  line L14 (-23.5, 7.5) -> (-38.5, 7.5)
  line L15 (-38.5, 7.5) -> (-38.5, 17.5)
  line L16 (-38.5, 17.5) -> (-23.5, 17.5)
  line L17 (-23.5, 17.5) -> (-23.5, 7.5)
  point P0 (-43, -25)
  dimension "d134" = 7.5
  dimension "d135" = 23.5
  dimension "d136" = 15
  dimension "d137" = 10
  constraints: 8 end point, 2 parallel, 1 horizontal, 1 perpendicular
  measures "d134" distance between parallel lines of L7 L16
  measures "d135" distance between parallel lines of L8 L17
  measures "d136" distance between parallel lines of L17 L15
  measures "d137" distance between parallel lines of L16 L14
extrude "Extrusion12" cut sketch "Sketch15" against normal up to surface (2.5 mm away) contours L14 L15 L16 L17
sketch "Sketch17" plane through (0, 0, 0) normal (0, 0, -1) x (-1, 0, 0)
  circle A0 centre (0, -40) radius 1.65 projected
  arc A1 (24.4212, -50) -> (27.86, -45.25) centre (22.86, -45.25) ccw projected
  line L0 (24.4212, -50) -> (21.2988, -50) projected
  arc A2 (17.86, -45.25) -> (21.2988, -50) centre (22.86, -45.25) ccw projected
  line L1 (17.86, -45.25) -> (17.86, 9.75) projected
  arc A3 (17.86, 9.75) -> (12.86, 14.75) centre (12.86, 9.75) ccw projected
  line L2 (12.86, 14.75) -> (4, 14.75) projected
  line L3 (4, 14.75) -> (4, -40) projected
  arc A4 (-4, -40) -> (4, -40) centre (0, -40) ccw projected
  line L4 (-4, -40) -> (-4, 14.75) projected
  line L5 (-4, 14.75) -> (-12.86, 14.75) projected
  arc A5 (-12.86, 14.75) -> (-17.86, 9.75) centre (-12.86, 9.75) ccw projected
  line L6 (-17.86, 9.75) -> (-17.86, -45.25) projected
  arc A6 (-21.2988, -50) -> (-17.86, -45.25) centre (-22.86, -45.25) ccw projected
  line L7 (-21.2988, -50) -> (-24.4212, -50) projected
  arc A7 (-27.86, -45.25) -> (-24.4212, -50) centre (-22.86, -45.25) ccw projected
  line L8 (-27.86, -45.25) -> (-27.86, 11.9507) projected
  arc A8 (-27.86, 11.9507) -> (-30.2465, 16.2132) centre (-32.86, 11.9507) ccw projected
  line L9 (-30.2465, 16.2132) -> (-40.5, 22.5) projected
  line L10 (-40.5, 22.5) -> (-43, 25) projected
  line L11 (-43, 25) -> (-43, 50) projected
  line L12 (-43, 50) -> (-40.5, 50) projected
  line L13 (-40.5, 50) -> (-13, 50) projected
  line L14 (-13, 32) -> (-13, 50) projected
  line L15 (-40.5, 32) -> (-13, 32) projected
  line L16 (-40.5, 34.5) -> (-40.5, 32) projected
  line L17 (-15.5, 34.5) -> (-40.5, 34.5) projected
  line L18 (-15.5, 47.5) -> (-15.5, 34.5) projected
  line L19 (-21.3291, 47.5) -> (-15.5, 47.5) projected
  arc A9 (-24.3909, 47.5) -> (-21.3291, 47.5) centre (-22.86, 44.92) ccw projected
  arc A10 (-21.3291, 47.5) -> (-24.3909, 47.5) centre (-22.86, 44.92) ccw projected
  line L20 (27.86, 11.9507) -> (27.86, -45.25) projected
  arc A11 (30.2465, 16.2132) -> (27.86, 11.9507) centre (32.86, 11.9507) ccw projected
  line L21 (39.996, 22.191) -> (30.2465, 16.2132) projected
  arc A12 (39.996, 22.191) -> (40.918, 22.918) centre (37.3825, 26.4536) ccw projected
  line L22 (43, 25) -> (40.918, 22.918) projected
  line L23 (43, 50) -> (43, 25) projected
  line L24 (40.5, 50) -> (43, 50) projected
  line L25 (13, 50) -> (40.5, 50) projected
  line L26 (13, 50) -> (13, 32) projected
  line L27 (13, 32) -> (40.5, 32) projected
  line L28 (40.5, 32) -> (40.5, 34.5) projected
  line L29 (40.5, 34.5) -> (15.5, 34.5) projected
  line L30 (15.5, 34.5) -> (15.5, 47.5) projected
  line L31 (21.3291, 47.5) -> (15.5, 47.5) projected
  arc A13 (21.3291, 47.5) -> (24.3909, 47.5) centre (22.86, 44.92) ccw projected
  line L32 (24.3909, 47.5) -> (40.5, 47.5) projected
  line L33 (40.5, 47.5) -> (40.5, 50) projected
  line L34 (-40.5, 50) -> (-40.5, 47.5) projected
  line L35 (-24.3909, 47.5) -> (-40.5, 47.5) projected
  line L36 (-13, 50) -> (13, 50) projected
  arc A14 (24.3909, 47.5) -> (21.3291, 47.5) centre (22.86, 44.92) ccw projected
  point P0 (0, 0)
hole "Hole5" at (22.86, -45.25, 0) at (-22.86, -45.25, 0) direction (0, 0, 1) diameter 3.3 depth 2.5
sketch "Sketch18" plane through (0, 0, 2.5) normal (0, 0, 1) x (1, 0, 0)
  circle A0 centre (-22.86, -45.25) radius 1.65 projected
  circle A1 centre (22.86, -45.25) radius 1.65 projected
  circle A2 centre (0, -40) radius 3 projected
  circle A3 centre (-22.86, 44.92) radius 1.65 projected
  circle A4 centre (22.86, 44.92) radius 1.65 projected
  arc A5 (-40.918, 22.918) -> (-39.996, 22.191) centre (-37.3825, 26.4536) ccw projected
  line L0 (-40.918, 22.918) -> (-43, 25) projected
  line L1 (-43, 25) -> (-40.5, 25) projected
  line L2 (-40.5, 25) -> (-40.5, 50) projected
  line L3 (-40.5, 50) -> (40.5, 50) projected
  line L4 (40.5, 50) -> (40.5, 25) projected
  line L5 (40.5, 25) -> (43, 25) projected
  line L6 (43, 25) -> (40.5, 22.5) projected
  line L7 (40.5, 22.5) -> (30.2465, 16.2132) projected
  arc A6 (30.2465, 16.2132) -> (27.86, 11.9507) centre (32.86, 11.9507) ccw projected
  line L8 (27.86, 11.9507) -> (27.86, -45.25) projected
  arc A7 (24.4212, -50) -> (27.86, -45.25) centre (22.86, -45.25) ccw projected
  line L9 (24.4212, -50) -> (21.2988, -50) projected
  arc A8 (17.86, -45.25) -> (21.2988, -50) centre (22.86, -45.25) ccw projected
  line L10 (17.86, -45.25) -> (17.86, 9.75) projected
  arc A9 (17.86, 9.75) -> (12.86, 14.75) centre (12.86, 9.75) ccw projected
  line L11 (12.86, 14.75) -> (4, 14.75) projected
  line L12 (4, 14.75) -> (4, -40) projected
  arc A10 (-4, -40) -> (4, -40) centre (0, -40) ccw projected
  line L13 (-4, -40) -> (-4, 14.75) projected
  line L14 (-4, 14.75) -> (-12.86, 14.75) projected
  arc A11 (-12.86, 14.75) -> (-17.86, 9.75) centre (-12.86, 9.75) ccw projected
  line L15 (-17.86, 9.75) -> (-17.86, -45.25) projected
  arc A12 (-21.2988, -50) -> (-17.86, -45.25) centre (-22.86, -45.25) ccw projected
  line L16 (-21.2988, -50) -> (-24.4212, -50) projected
  arc A13 (-27.86, -45.25) -> (-24.4212, -50) centre (-22.86, -45.25) ccw projected
  line L17 (-27.86, -45.25) -> (-27.86, 11.9507) projected
  arc A14 (-27.86, 11.9507) -> (-30.2465, 16.2132) centre (-32.86, 11.9507) ccw projected
  line L18 (-30.2465, 16.2132) -> (-39.996, 22.191) projected
  line L19 (-43, 25) -> (-43, 50) projected
  line L20 (-43, 50) -> (-40.5, 50) projected
  line L21 (40.5, 50) -> (43, 50) projected
  line L22 (43, 50) -> (43, 25) projected
  circle A15 centre (-22.86, -45.25) radius 5
  circle A16 centre (22.86, -45.25) radius 5
  point P0 (0, 0)
  constraints: 2 centre point, 2 coincident, 2 concentric
extrude "Extrusion14" add sketch "Sketch18" against normal up to surface (2.5 mm away) contours L16 A15 | A16 L9
equation "\"d20\" = d19"
equation "\"d68\" = d69"
equation "\"d70\" = d68"
equation "\"d71\" = d69"
equation "\"d75\" = d74"
equation "\"d82\" = d83"
equation "\"d89\" = d88"
equation "\"d108\" = d109"
equation "\"d110\" = d109"
body "Solid1"
